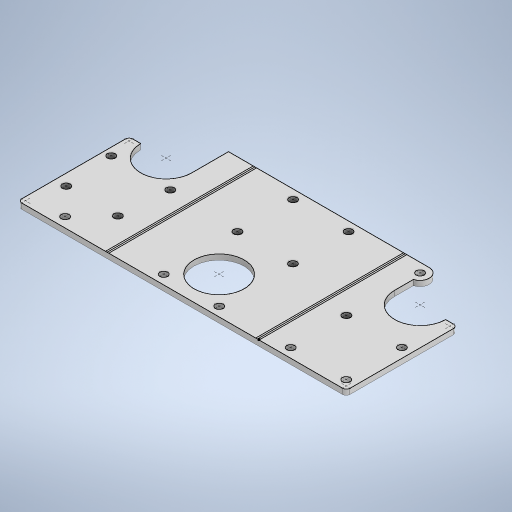
# Autodesk Inventor part: axis_3_top_frame
Saved by Autodesk Inventor 2024.2 (Build 282272000, 272)
## iProperties
Created: 2024-01-02
Part Number: axis_3_top_frame
Material: Generic
Document SubType Name: Modeling
Designer: chanh
Density: 1 g/cm^3
Appearance: Default
Author: chanh
Autodesk Inventor part; units mm, degrees
ref_plane "YZ Plane" through (0, 0, 0) normal (1, 0, 0) x (0, 1, 0)
ref_plane "XZ Plane" through (0, 0, 0) normal (0, 1, 0) x (-1, 0, 0)
ref_plane "XY Plane" through (0, 0, 0) normal (0, 0, 1) x (1, 0, 0)
sketch "Sketch1" plane through (0, 0, 0) normal (0, 1, 0) x (-1, 0, 0)
  line L0 (87.8296, -40.1) -> (87.8296, 0)
  line L1 (128.6089, 0) -> (128.6089, -40.1)
  circle A0 centre (81.285, -37.6) radius 1.05
  circle A1 centre (66.235, -17.6) radius 1.05
  circle A2 centre (81.285, -17.6) radius 1.05
  circle A3 centre (66.235, -2.5) radius 1.05
  circle A4 centre (81.285, -2.5) radius 1.05
  circle A5 centre (115.7443, -37.6) radius 1.05
  circle A6 centre (100.6943, -37.6) radius 1.05
  circle A7 centre (115.7443, -22.5) radius 1.05
  circle A8 centre (100.6943, -22.5) radius 1.05
  circle A9 centre (115.7443, -2.5) radius 1.05
  circle A10 centre (100.6943, -2.5) radius 1.05
  circle A11 centre (108.2193, -10) radius 6.8
  circle A12 centre (142.6786, -2.68) radius 1.05
  circle A13 centre (149.6786, -9.98) radius 1.05
  circle A14 centre (135.6786, -9.98) radius 1.05
  circle A15 centre (150.6786, -23.2) radius 1.05
  circle A16 centre (134.6786, -23.2) radius 1.05
  arc A17 (64.69, 0) -> (63.69, -1) centre (64.69, -1) ccw
  arc A18 (152.7486, -1) -> (151.7486, 0) centre (151.7486, -1) ccw
  line L2 (152.7486, -29.1) -> (152.7486, -1)
  arc A19 (151.7486, -30.1) -> (152.7486, -29.1) centre (151.7486, -29.1) ccw
  line L3 (151.7486, -30.1) -> (149.5786, -30.1)
  arc A20 (149.5786, -30.1) -> (135.7786, -30.1) centre (142.6786, -30.1) ccw
  line L4 (135.7786, -30.1) -> (135.7786, -40.1)
  line L5 (81.285, -40.1) -> (135.7786, -40.1)
  arc A21 (80.66, -35.1794) -> (81.285, -40.1) centre (81.285, -37.6) ccw
  line L6 (80.66, -35.1794) -> (80.66, -30.1)
  arc A22 (80.66, -30.1) -> (66.86, -30.1) centre (73.76, -30.1) ccw
  line L7 (66.86, -30.1) -> (64.69, -30.1)
  arc A23 (63.69, -29.1) -> (64.69, -30.1) centre (64.69, -29.1) ccw
  line L8 (63.69, -1) -> (63.69, -29.1)
  line L9 (151.7486, 0) -> (64.69, 0)
  line L10 (129.0586, -40.1) -> (129.0586, 0)
  line L11 (128.1593, 0) -> (128.1593, -40.1)
  line L12 (88.2793, -40.1) -> (88.2793, 0)
  line L13 (87.38, 0) -> (87.38, -40.1)
  constraints: 28 end point, 24 centre point, 14 point on circle, 12 point on line, 10 vertical, 4 horizontal, 75 other
extrude "Extrusion1" add sketch "Sketch1" against normal blind 1.5
body "Solid2"
